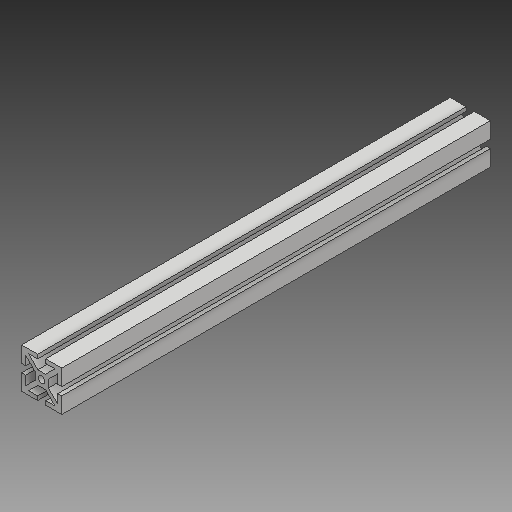
# Autodesk Inventor part: item_30x30_32cm
Saved by Autodesk Inventor 2018 (Build 220112000, 112)
## iProperties
Created: 2020-03-29
Part Number: item_30x30_32cm
Material: Generisch
Document SubType Name: Modeling
Designer: wepet
Density: 1 g/cm^3
Appearance: Vorgabe
Description: Aluprofil 30x30 - 32cm
Mass: 0.144371 g
Surface Area: 9.46504 cm^2
Volume: 0.144371 cm^3
Author: wepet
Autodesk Inventor part; units mm, degrees
ref_plane "YZ Plane" through (0, 0, 0) normal (1, 0, 0) x (0, 1, 0)
ref_plane "XZ Plane" through (0, 0, 0) normal (0, 1, 0) x (-1, 0, 0)
ref_plane "XY Plane" through (0, 0, 0) normal (0, 0, 1) x (1, 0, 0)
sketch "Skizze1" plane through (0, 0, 0) normal (0, 1, 0) x (-1, 0, 0)
  line L0 (0, 0) -> (3, 0) construction
  line L1 (3, 0) -> (3, -3) construction
  line L2 (3, -3) -> (0, -3) construction
  line L3 (0, -3) -> (0, 0) construction
  line L4 (3, -1.5) -> (0, -1.5) construction
  line L5 (1.5, -3) -> (1.5, 0) construction
  circle A0 centre (1.5, -1.5) radius 0.25
  line L6 (2, -1) -> (1, -1) construction
  line L7 (1, -1) -> (1, -2) construction
  line L8 (1, -2) -> (2, -2) construction
  line L9 (2, -2) -> (2, -1) construction
  line L10 (1.5, -1) -> (1.5, -2) construction
  line L11 (2, -1.5) -> (1, -1.5) construction
  line L12 (3, -1.2) -> (0, -1.2) construction
  line L13 (1.2, 0) -> (1.2, -3) construction
  line L14 (0, -1.8) -> (3, -1.8) construction
  line L15 (1.8, 0) -> (1.8, -3) construction
  line L16 (2.7, -2.7) -> (2.7, -0.3) construction
  line L17 (2.7, -0.3) -> (0.3, -0.3) construction
  line L18 (0.3, -0.3) -> (0.3, -2.7) construction
  line L19 (0.3, -2.7) -> (2.7, -2.7) construction
  line L20 (2.7, -0.3) -> (0.3, -2.7) construction
  line L21 (2.7, -2.7) -> (0.3, -0.3) construction
  line L22 (2.7, -0.5121) -> (0.5121, -2.7) construction
  line L23 (0.3, -2.4879) -> (2.4879, -0.3) construction
  line L24 (0.5121, -0.3) -> (2.7, -2.4879) construction
  line L25 (2.4879, -2.7) -> (0.3, -0.5121) construction
  line L26 (3, 0) -> (3, -1.2)
  line L27 (3, -1.2) -> (2.7, -1.2)
  line L28 (2.7, -1.2) -> (2.7, -0.5121)
  line L29 (2.7, -0.5121) -> (2, -1.2121)
  line L30 (2, -1.2121) -> (2, -1.7879)
  line L31 (2, -1.7879) -> (2.7, -2.4879)
  line L32 (2.7, -2.4879) -> (2.7, -1.8)
  line L33 (2.7, -1.8) -> (3, -1.8)
  line L34 (3, -3) -> (3, -1.8)
  line L35 (3, -3) -> (1.8, -3)
  line L36 (1.8, -3) -> (1.8, -2.7)
  line L37 (1.8, -2.7) -> (2.4879, -2.7)
  line L38 (1.7879, -2) -> (2.4879, -2.7)
  line L39 (1.2121, -2) -> (1.7879, -2)
  line L40 (1.2121, -2) -> (0.5121, -2.7)
  line L41 (0.5121, -2.7) -> (1.2, -2.7)
  line L42 (1.2, -2.7) -> (1.2, -3)
  line L43 (1.2, -3) -> (0, -3)
  line L44 (0, -3) -> (0, -1.8)
  line L45 (0.3, -1.8) -> (0, -1.8)
  line L46 (0.3, -1.8) -> (0.3, -2.4879)
  line L47 (0.3, -2.4879) -> (1, -1.7879)
  line L48 (1, -1.7879) -> (1, -1.2121)
  line L49 (1, -1.2121) -> (0.3, -0.5121)
  line L50 (0.3, -0.5121) -> (0.3, -1.2)
  line L51 (0.3, -1.2) -> (0, -1.2)
  line L52 (0, -1.2) -> (0, 0)
  line L53 (0, 0) -> (1.2, 0)
  line L54 (1.2, 0) -> (1.2, -0.3)
  line L55 (1.2, -0.3) -> (0.5121, -0.3)
  line L56 (0.5121, -0.3) -> (1.2121, -1)
  line L57 (1.2121, -1) -> (1.7879, -1)
  line L58 (1.7879, -1) -> (2.4879, -0.3)
  line L59 (2.4879, -0.3) -> (1.8, -0.3)
  line L60 (1.8, -0.3) -> (1.8, 0)
  line L61 (1.8, 0) -> (3, 0)
  dimension "d0" = 3
  dimension "d1" = 3
  dimension "d2" = 0.5
  dimension "d3" = 1
  dimension "d4" = 1
  dimension "d5" = 1.2
  dimension "d6" = 1.2
  dimension "d7" = 1.2
  dimension "d8" = 1.2
  dimension "d9" = 0.3
  dimension "d10" = 0.15
  dimension "d11" = 0.15
  dimension "d12" = 0.15
  dimension "d13" = 0.15
  constraints: 124 end point, 48 point on line, 15 collinear, 13 perpendicular, 11 midpoint, 10 parallel, 2 horizontal, 1 centre point, 3 other
  measures "d0" distance of L1.end L2.end
  measures "d1" distance of L0.end L1.end
  measures "d2" diameter of A0
  measures "d3" distance of L8.end L6.start
  measures "d4" distance of L6.start L6.end
  measures "d5" distance between parallel lines of L1 L15
  measures "d6" distance between parallel lines of L3 L13
  measures "d7" distance between parallel lines of L2 L14
  measures "d8" distance between parallel lines of L0 L12
  measures "d9" distance between parallel lines of L1 L16
  measures "d10" distance between parallel lines of L24 L21
  measures "d11" distance between parallel lines of L21 L25
  measures "d12" distance between parallel lines of L20 L22
  measures "d13" distance between parallel lines of L20 L23
extrude "Extrusion1" add sketch "Skizze1" along normal blind 32
